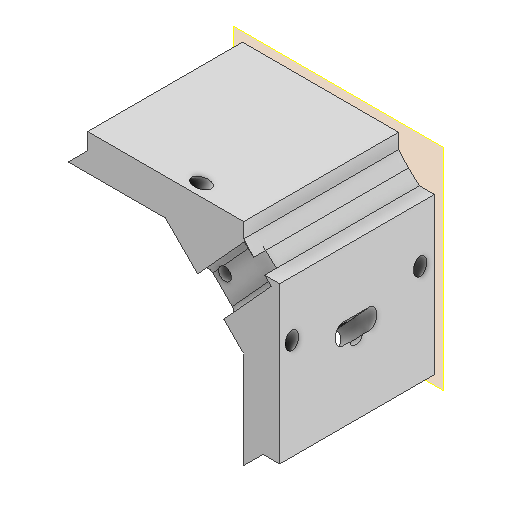
# Autodesk Inventor part: 20_Cube_Insert_Kinematic_Mirror_45_pro_v3
Saved by Autodesk Inventor 2022 (Build 260153000, 153)
## iProperties
Created: 2022-01-05
Part Number: 20_Cube_Insert_Kinematic_Mirror_45_pro_v3
Material: Generisch
Document SubType Name: Modeling
Designer: diederichbenedict
Density: 1 g/cm^3
Appearance: Vorgabe
Author: diederichbenedict
Autodesk Inventor part; units mm, degrees
ref_plane "YZ Plane" through (0, 0, 0) normal (1, 0, 0) x (0, 1, 0)
ref_plane "XZ Plane" through (0, 0, 0) normal (0, 1, 0) x (-1, 0, 0)
ref_plane "XY Plane" through (0, 0, 0) normal (0, 0, 1) x (1, 0, 0)
ref_plane "Arbeitsebene1" through (0, 0, 0) normal (0, 0, 1) x (1, 0, 0)
sketch "Skizze1" plane through (0, 0, 0) normal (0, 0, 1) x (1, 0, 0)
  arc A0 (24.9, 22.9) -> (22.9, 24.9) centre (22.9, 22.9) ccw projected
  line L0 (22.9, 24.9) -> (-17.02, 24.9) projected
  line L1 (-17.02, 24.9) -> (-17.02, 21.2686) projected
  line L2 (-17.02, 21.2) -> (17.02, 21.2) projected
  line L3 (-21.2698, 17.02) -> (-17.02, 17.02) projected
  line L4 (21.2698, 17.02) -> (21.2698, -17.02) projected
  line L5 (21.2698, -17.02) -> (17.02, -17.02) projected
  line L6 (24.9, -17.02) -> (24.9, 22.9) projected
  line L7 (23.75, 23.25) -> (23.75, 18.15) projected
  arc A1 (23.25, 17.65) -> (23.75, 18.15) centre (23.25, 18.15) ccw projected
  line L8 (23.25, 17.65) -> (20.8937, 17.65) projected
  arc A2 (20.5239, 17.8134) -> (20.8937, 17.65) centre (20.8937, 18.15) ccw projected
  line L9 (20.5239, 17.8134) -> (17.7803, 20.8273) projected
  arc A3 (17.65, 21.1639) -> (17.7803, 20.8273) centre (18.15, 21.1639) ccw projected
  line L10 (17.65, 21.1639) -> (17.65, 23.25) projected
  arc A4 (18.15, 23.75) -> (17.65, 23.25) centre (18.15, 23.25) ccw projected
  line L11 (18.15, 23.75) -> (23.25, 23.75) projected
  arc A5 (23.75, 23.25) -> (23.25, 23.75) centre (23.25, 23.25) ccw projected
  line L12 (-17.02, 24.9) -> (17.0606, 24.9)
  line L13 (17.0606, 24.9) -> (17.0606, 21.9)
  line L14 (17.0606, 21.9) -> (-17.02, 21.9)
  line L15 (34.79, 34.79) -> (-34.79, -34.79)
  line L16 (17.0606, 21.9) -> (17.0606, 17.0606)
  line L17 (13.0606, 21.9) -> (13.0606, 13.0606)
  line L18 (17.0606, 17.0606) -> (13.0606, 13.0606)
  line L19 (17.02, 17.02) -> (-17.02, 17.02) projected
  line L20 (17.02, 21.2) -> (17.02, 17.02) projected
  line L21 (-17.02, 21.2) -> (17.02, 21.2) projected
  line L22 (-17.02, 24.9) -> (-17.02, 21.2686) projected
  line L23 (-21.2711, 17.02) -> (-17.02, 21.2686) projected
  line L24 (17.02, 17.02) -> (21.2698, 17.02) projected
  line L25 (-17.02, 21.9) -> (-13.02, 21.9)
  line L26 (-13.02, 21.9) -> (-13.02, 17.02)
  line L27 (-13.02, 17.02) -> (-17.02, 17.02)
  line L28 (-17.02, 17.02) -> (-17.02, 21.9)
  line L29 (-17.02, 21.2686) -> (-21.2711, 17.02)
  line L30 (-21.2711, 17.02) -> (-17.02, 17.02)
  line L31 (-4.9294, 21.9) -> (21.2698, -4.2993)
  line L32 (21.2698, 2.7718) -> (2.1416, 21.9)
  line L33 (12.0208, 12.0208) -> (8.4853, 8.4853)
  line L34 (-17.02, 17.02) -> (-17.02, 21.2) projected
  line L35 (-17.02, -21.2) -> (-17.02, -17.02) projected
  line L36 (-21.2698, -17.02) -> (-21.2698, 17.02) projected
  line L37 (-17.02, 17.02) -> (-17.02, 21.2) projected
  line L38 (17.02, 21.2) -> (17.02, 17.02) projected
  line L39 (17.02, 17.02) -> (21.2698, 17.02) projected
  line L40 (17.02, -17.02) -> (17.02, -21.2) projected
  line L41 (17.02, -21.2) -> (-17.02, -21.2) projected
  line L42 (-20.8273, -17.7803) -> (-17.8134, -20.5239) projected
  arc A6 (-17.65, -20.8937) -> (-17.8134, -20.5239) centre (-18.15, -20.8937) ccw projected
  line L43 (-17.65, -20.8937) -> (-17.65, -23.25) projected
  arc A7 (-18.15, -23.75) -> (-17.65, -23.25) centre (-18.15, -23.25) ccw projected
  line L44 (-18.15, -23.75) -> (-23.25, -23.75) projected
  arc A8 (-23.75, -23.25) -> (-23.25, -23.75) centre (-23.25, -23.25) ccw projected
  line L45 (-23.75, -23.25) -> (-23.75, -18.15) projected
  arc A9 (-23.25, -17.65) -> (-23.75, -18.15) centre (-23.25, -18.15) ccw projected
  line L46 (-23.25, -17.65) -> (-21.1639, -17.65) projected
  arc A10 (-20.8273, -17.7803) -> (-21.1639, -17.65) centre (-21.1639, -18.15) ccw projected
  line L47 (-21.2711, 17.02) -> (-17.02, 21.2686) projected
  line L48 (-21.2711, 17.02) -> (-24.9, 17.02) projected
  line L49 (-24.9, 17.02) -> (-24.9, -22.9) projected
  arc A11 (-24.9, -22.9) -> (-22.9, -24.9) centre (-22.9, -22.9) ccw projected
  line L50 (-22.9, -24.9) -> (17.02, -24.9) projected
  line L51 (17.02, -24.9) -> (17.02, -21.2686) projected
  line L52 (21.2711, -17.02) -> (17.02, -21.2686) projected
  line L53 (21.2711, -17.02) -> (24.9, -17.02) projected
  line L54 (-17.02, -21.2) -> (-17.02, -17.02) projected
  line L55 (-17.02, -17.02) -> (-21.2698, -17.02) projected
  line L56 (-21.2698, -17.02) -> (-21.2698, 17.02) projected
  line L57 (-17.02, 17.02) -> (-17.02, 21.2) projected
  line L58 (-17.02, 21.2) -> (17.02, 21.2) projected
  line L59 (17.02, 21.2) -> (17.02, 17.02) projected
  line L60 (21.2698, 17.02) -> (21.2698, -17.02) projected
  line L61 (21.2698, -17.02) -> (17.02, -17.02) projected
  line L62 (17.02, -17.02) -> (17.02, -21.2) projected
  line L63 (17.02, -21.2) -> (-17.02, -21.2) projected
  line L64 (-20.8273, -17.7803) -> (-17.8134, -20.5239) projected
  arc A12 (-17.65, -20.8937) -> (-17.8134, -20.5239) centre (-18.15, -20.8937) ccw projected
  line L65 (-17.65, -20.8937) -> (-17.65, -23.25) projected
  arc A13 (-18.15, -23.75) -> (-17.65, -23.25) centre (-18.15, -23.25) ccw projected
  line L66 (-18.15, -23.75) -> (-23.25, -23.75) projected
  arc A14 (-23.75, -23.25) -> (-23.25, -23.75) centre (-23.25, -23.25) ccw projected
  line L67 (-23.75, -23.25) -> (-23.75, -18.15) projected
  arc A15 (-23.25, -17.65) -> (-23.75, -18.15) centre (-23.25, -18.15) ccw projected
  line L68 (-23.25, -17.65) -> (-21.1639, -17.65) projected
  arc A16 (-20.8273, -17.7803) -> (-21.1639, -17.65) centre (-21.1639, -18.15) ccw projected
  line L69 (23.75, 23.25) -> (23.75, 18.15) projected
  arc A17 (23.25, 17.65) -> (23.75, 18.15) centre (23.25, 18.15) ccw projected
  line L70 (23.25, 17.65) -> (20.8937, 17.65) projected
  arc A18 (20.5239, 17.8134) -> (20.8937, 17.65) centre (20.8937, 18.15) ccw projected
  line L71 (20.5239, 17.8134) -> (17.7803, 20.8273) projected
  arc A19 (17.65, 21.1639) -> (17.7803, 20.8273) centre (18.15, 21.1639) ccw projected
  line L72 (17.65, 21.1639) -> (17.65, 23.25) projected
  arc A20 (18.15, 23.75) -> (17.65, 23.25) centre (18.15, 23.25) ccw projected
  line L73 (18.15, 23.75) -> (23.25, 23.75) projected
  arc A21 (23.75, 23.25) -> (23.25, 23.75) centre (23.25, 23.25) ccw projected
  arc A22 (24.9, 22.9) -> (22.9, 24.9) centre (22.9, 22.9) ccw projected
  line L74 (22.9, 24.9) -> (-17.02, 24.9) projected
  line L75 (-21.2711, 17.02) -> (-24.9, 17.02) projected
  line L76 (-24.9, 17.02) -> (-24.9, -22.9) projected
  arc A23 (-24.9, -22.9) -> (-22.9, -24.9) centre (-22.9, -22.9) ccw projected
  line L77 (-22.9, -24.9) -> (17.02, -24.9) projected
  line L78 (17.02, -24.9) -> (17.02, -21.2686) projected
  line L79 (21.2711, -17.02) -> (17.02, -21.2686) projected
  line L80 (21.2711, -17.02) -> (24.9, -17.02) projected
  line L81 (24.9, -17.02) -> (24.9, 22.9) projected
  line L82 (19.2323, 19.2323) -> (17.0606, 21.6178)
  line L83 (-17.02, -17.02) -> (-21.2698, -17.02) projected
  line L84 (-21.2698, 17.02) -> (-17.02, 17.02) projected
  point P0 (0, 0)
  point P1 (17.0606, 24.9)
  point P2 (-16.97, 16.97)
  point P3 (-13.02, 17.02)
  point P4 (-13.02, 21.2)
  point P5 (13.0606, 21.2)
  point P6 (2.8416, 21.2)
  point P7 (-4.2294, 21.2)
  point P8 (13.0606, 17.02)
  point P9 (16.97, 21.2)
  point P10 (-16.97, 17.02)
  point P11 (-17.02, 20.7)
  point P12 (13.0606, 21.2)
  point P13 (-16.97, 21.2)
  point P14 (-17.02, 21.9)
  point P15 (19.2323, 19.2323)
  point P16 (23.6036, 23.6036)
  point P17 (24.3142, 24.3142)
  point P18 (16.97, 17.02)
  point P19 (7.0216, 17.02)
  point P20 (-0.0494, 17.02)
  point P21 (-17.02, 17.02)
  dimension "d3" = 4
  dimension "d6" = 4
  dimension "d9" = 0
  dimension "d11" = 5
  dimension "d35" = 0
  constraints: 32 end point, 11 point on line, 4 parallel, 2 collinear, 2 horizontal, 2 perpendicular, 1 vertical, 11 other
  measures "d3" distance between parallel lines of L16 L17
  measures "d6" distance of L26.end L27.end
  measures "d9" distance between parallel lines of L23 L29
  measures "d11" distance between parallel lines of L32 L31
  measures "d35" distance between parallel lines of L9 L82
extrude "Extrusion1" add sketch "Skizze1" along normal blind 33.8 contours L13 L14 L1 L0 | L15 L16 L82 L9 | L16 L15 L20 L2 L17 L14 | L31 L19 L32 L15 | L14 L26 L2 L28 L1 | L17 L2 L32 L14 | L15 L17 L19 | L19 L17 L2 L20 | L32 L19 L17 L15 | L31 L2 L32 L19 | L19 L26 L2 L31 | L28 L3 L23 | L14 L31 L2 L26 | L32 L2 L31 L14 | L17 L19 L32 L2 | L19 L28 L2 L26
mirror "Spiegeln1" about plane through (8.4853, 8.4853, 0) normal (0.7071, -0.7071, 0) of "Extrusion1"
sketch "Skizze2" plane through (17.6463, 20.9745, 0) normal (0.7395, 0.6732, 0) x (-0.6732, 0.7395, 0)
  circle A0 centre (-16.6729, 31.13) radius 1.45
  circle A1 centre (-16.6729, 3.13) radius 1.45
  circle A2 centre (11.3271, 31.13) radius 1.45
  point P0 (-3.6312, 0)
  dimension "d36" = 2.9
  dimension "d37" = 2.9
  dimension "d38" = 2.9
  constraints: 3 centre point, 3 coincident
  measures "d36" diameter of A0
  measures "d37" diameter of A1
  measures "d38" diameter of A2
sketch "Skizze3" plane through (17.2397, 21.0462, 0) normal (0.6732, 0.7395, 0) x (-0.7395, 0.6732, 0)
  line L0 (-17.8955, 20.13) -> (-17.8955, 14.13) projected
  line L1 (-20.8922, 14.13) -> (-20.8922, 20.13) projected
  line L2 (-0.9142, 31.21) -> (-6.9076, 31.21) projected
  line L3 (-6.9076, 34.21) -> (-0.9142, 34.21) projected
  line L4 (13.0291, 42.03) -> (-20.8922, 42.03) projected
  line L5 (-20.8922, 42.03) -> (-20.8922, 38.4552) projected
  line L6 (-20.8922, 38.4552) -> (-25.2126, 34.13) projected
  line L7 (-25.2126, 34.13) -> (-28.7835, 34.13) projected
  line L8 (-28.7835, 34.13) -> (-28.7835, 0.13) projected
  line L9 (-28.7835, 0.13) -> (-25.2126, 0.13) projected
  line L10 (-25.2126, 0.13) -> (-20.8922, -4.1952) projected
  line L11 (-20.8922, -4.1952) -> (-20.8922, -7.77) projected
  line L12 (-20.8922, -7.77) -> (13.0704, -7.77) projected
  line L13 (13.0704, -7.77) -> (13.0704, -4.1952) projected
  line L14 (13.0704, -4.1952) -> (17.3909, 0.13) projected
  line L15 (17.3909, 0.13) -> (20.9618, 0.13) projected
  line L16 (20.9618, 0.13) -> (20.9618, 34.13) projected
  line L17 (20.9618, 34.13) -> (17.3909, 34.13) projected
  line L18 (17.3909, 34.13) -> (13.0291, 38.4966) projected
  line L19 (13.0291, 38.4966) -> (13.0291, 42.03) projected
  ellipse E0 centre (-19.3938, 14.13) end of major axis (-19.3938, 15.63) minor radius 1.4984 (-20.8922, 14.13) -> (-17.8955, 14.13) ccw projected
  ellipse E1 centre (-19.3938, 20.13) end of major axis (-19.3938, 18.63) minor radius 1.4984 (-17.8955, 20.13) -> (-20.8922, 20.13) ccw projected
  ellipse E2 centre (-6.9076, 32.71) end of major axis (-6.9076, 34.21) minor radius 1.4984 (-6.9076, 34.21) -> (-6.9076, 31.21) ccw projected
  ellipse E3 centre (-0.9142, 32.71) end of major axis (-0.9142, 31.21) minor radius 1.4984 (-0.9142, 31.21) -> (-0.9142, 34.21) ccw projected
  ellipse E4 centre (-17.8955, 31.13) end of major axis (-17.8955, 34.38) minor radius 3.2464 projected
  ellipse E5 centre (-3.9109, 17.13) end of major axis (-3.9109, 20.38) minor radius 3.2464 projected
  ellipse E6 centre (10.0737, 31.13) end of major axis (10.0737, 34.38) minor radius 3.2464 projected
  ellipse E7 centre (-17.8955, 3.13) end of major axis (-17.8955, 6.38) minor radius 3.2464 projected
  point P0 (-1.4194, 0)
  constraints: 4 other
extrude "Extrusion2" cut sketch "Skizze3" against normal blind 33.8 contours L0 E0 L1 E1 | L2 E2 L3 E3
sketch "Skizze4" plane through (0, 0, 33.8) normal (0, 0, 1) x (1, 0, 0)
  line L0 (22.3477, 16.3962) -> (11.972, 4.9986) projected
  line L1 (17.9157, 20.4308) -> (7.7294, 9.2412) projected
  circle A0 centre (10.3701, 10.3701) radius 1.4
  line L2 (19.2323, 19.2323) -> (21.6178, 17.0606) projected
  line L3 (19.2323, 19.2323) -> (17.9157, 20.4308) projected
  line L4 (11.972, 4.9986) -> (7.7294, 9.2412) projected
  line L5 (22.3477, 16.3962) -> (21.6178, 17.0606) projected
  point P0 (0, 0)
  dimension "d26" = 2.8
  constraints: 1 centre point
  measures "d26" diameter of A0
extrude "Extrusion3" cut sketch "Skizze4" against normal blind 20 contours A0 L1 | L1 A0
sketch "Skizze5" plane through (24.9, -16.97, 33.8) normal (1, 0, 0) x (0, 0, -1)
  line L0 (0, 34.0306) -> (0, -0.05) projected
  line L1 (33.8, 34.0306) -> (33.8, -0.05) projected
  line L2 (19.67, 15.5558) -> (13.67, 15.5558) projected
  circle A0 centre (16.67, 15.5558) radius 1.4
  line L3 (33.8, -0.05) -> (0, -0.05) projected
  line L4 (33.8, 34.0306) -> (0, 34.0306) projected
  point P0 (33.8, 16.97)
  dimension "d29" = 2.8
  constraints: 1 centre point, 1 midpoint
  measures "d29" diameter of A0
extrude "Extrusion4" cut sketch "Skizze5" against normal blind 20 contours A0 L2 | L2 A0
extrude "Extrusion6" cut sketch "Skizze2" against normal through all
